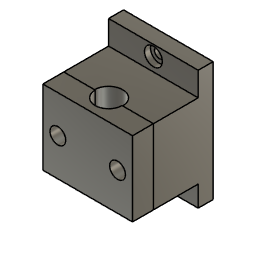
Needle holder v7 (Autodesk Fusion 360 design; units mm, degrees)
Autodesk Fusion 360 part; units mm, degrees
sketch "Sketch1" plane through (0, 0, 0) normal (0, 1, 0) x (1, 0, 0)
  line L0 (0, 0) -> (30, 0)
  line L1 (30, 0) -> (30, -40)
  line L2 (30, -40) -> (0, -40)
  line L3 (0, -40) -> (0, 0)
  circle A0 centre (15, -3.5) radius 1.65
  circle A1 centre (15, -36.5) radius 1.65
  dimension "d1" = 30
  dimension "d2" = 40
  dimension "d3" = 3.3
  dimension "d4" = 3.3
  dimension "d5" = 15
  dimension "d6" = 15
  dimension "d7" = 3.5
  dimension "d8" = 3.5
  constraint horizontal L0
  constraint vertical L1
  constraint horizontal L2
  constraint vertical L3
  constraint coincident L0.start L3.end
  measures "d1" distance of L0.start L0.end
  measures "d2" distance of L0.start L2.end
  measures "d3" diameter of A0
  measures "d4" diameter of A1
  measures "d5" distance of L3 A1.centre
  measures "d6" distance of L3 A0.centre
  measures "d7" distance of L2 A1.centre
  measures "d8" distance of L0 A0.centre
extrude "Extrude1" add sketch "Sketch1" along normal blind 5 makes body 1
sketch "Sketch2" plane through (0, 0, 0) normal (0, -1, 0) x (1, 0, 0)
  circle A0 centre (15, 3.5) radius 1.65
  circle A1 centre (15, 36.5) radius 1.65
  line L0 (30, 40) -> (0, 40)
  line L1 (0, 40) -> (0, 0)
  line L2 (0, 0) -> (30, 0)
  line L3 (30, 0) -> (30, 40)
  line L4 (0, 32) -> (30, 32)
  line L5 (30, 32) -> (30, 7)
  line L6 (30, 7) -> (0, 7)
  line L7 (0, 7) -> (0, 32)
  dimension "d11" = 8
  constraint horizontal L4
  constraint vertical L5
  constraint horizontal L6
  constraint vertical L7
  constraint coincident L3 L5.end
  constraint coincident L1 L4.start
  measures "d11" distance of L0 L4
extrude "Extrude2" add sketch "Sketch2" along normal blind 15 contours L1 L3 L4 L5 L6 L7 bodies 1
sketch "Sketch3" plane through (0, 0, 32) normal (0, 0, 1) x (-1, 0, 0)
  line L0 (-30, 0) -> (0, 0)
  line L1 (0, 0) -> (0, 15)
  line L2 (0, 15) -> (-30, 15)
  line L3 (-30, 15) -> (-30, 0)
  circle A0 centre (-15, 15) radius 4.7245
  dimension "d14" = 9.449
  constraint midpoint L2 A0.centre
  measures "d14" diameter of A0
extrude "Extrude3" cut sketch "Sketch3" against normal blind 25 contours L2 A0 picked at (-16.3012, 14.1129) bodies 1
ref_plane "WorkPlane1" through (15, -7.5, 20.8) normal (0, 0, 1) x (-1, 0, 0)
sketch "Sketch4" plane through (0, 0, 20.8) normal (0, 0, 1) x (1, 0, 0)
  circle A0 centre (15, -15) radius 5.7785
  dimension "d18" = 11.557
  measures "d18" diameter of A0
extrude "Extrude4" cut sketch "Sketch4" against normal blind 11.227 bodies 1
sketch "Sketch5" plane through (0, -15, 0) normal (0, -1, 0) x (1, 0, 0)
  line L0 (19.7245, 20.8) -> (20.7785, 20.8)
  line L1 (20.7785, 20.8) -> (20.7785, 9.573)
  line L2 (20.7785, 9.573) -> (19.7245, 9.573)
  line L3 (19.7245, 9.573) -> (19.7245, 7)
  line L4 (19.7245, 7) -> (30, 7)
  line L5 (30, 7) -> (30, 32)
  line L6 (30, 32) -> (19.7245, 32)
  line L7 (19.7245, 32) -> (19.7245, 20.8)
  circle A0 centre (25, 19.5) radius 2.5
  circle A1 centre (5, 19.5) radius 2.5
  line L8 (10.2755, 32) -> (0, 32)
  line L9 (0, 32) -> (0, 7)
  dimension "d21" = 5
  dimension "d22" = 5
  dimension "d23" = 12.5
  dimension "d24" = 12.5
  dimension "d25" = 5
  dimension "d26" = 5
  measures "d21" diameter of A0
  measures "d22" diameter of A1
  measures "d23" distance of A1.centre L8
  measures "d24" distance of L4 A0.centre
  measures "d25" distance of L5 A0.centre
  measures "d26" distance of A1.centre L9
extrude "Extrude5" cut sketch "Sketch5" against normal blind 5 contours A0 | A1 bodies 1
thread "Thread1" "ISO Metric profile 5.0 M5x0.8 6H" major diameter 5.12 minor diameter 4.234 pitch 0.8 angle 60 modelled right hand crest width 0.2219 on face at (7.4969, -11.6667, 19.3754) crest through (7.117, -14.8, 19.5) on bodies 1
thread "Thread2" "ISO Metric profile 5.0 M5x0.8 6H" major diameter 5.12 minor diameter 4.234 pitch 0.8 angle 60 modelled right hand crest width 0.2219 on face at (27.4969, -11.6667, 19.3754) crest through (27.117, -14.8, 19.5) on bodies 1
box "BoxPrimitive1" add length 25 width 30 height 7 placed x (0, 0, 1) y (-1, 0, 0) z (0, -1, 0) at (30, -15, 12.5) separate body makes body 2
sketch "Sketch9" plane through (0, 0, 37.5) normal (0, 0, 1) x (-1, 0, 0)
  line L0 (-30, 22) -> (-30, 15)
  line L1 (-30, 15) -> (0, 15)
  line L2 (0, 15) -> (0, 22)
  line L3 (0, 22) -> (-30, 22)
  circle A0 centre (-15, 15) radius 4.5
  dimension "d38" = 9
  constraint midpoint L1 A0.centre
  measures "d38" diameter of A0
extrude "Extrude6" cut sketch "Sketch9" against normal blind 25 contours L1 A0 picked at (-16.4501, 15.6657) bodies 2
ref_plane "WorkPlane2" through (15, -18.5, 26.3) normal (0, 0, 1) x (0, 1, 0)
sketch "Sketch10" plane through (0, 0, 26.3) normal (0, 0, 1) x (1, 0, 0)
  circle A0 centre (15, -15) radius 5.7785
  dimension "d42" = 11.557
  measures "d42" diameter of A0
extrude "Extrude7" cut sketch "Sketch10" against normal blind 11.227 bodies 2
sketch "Sketch11" plane through (0, -22, 0) normal (0, -1, 0) x (1, 0, 0)
  line L0 (30, 37.5) -> (0, 37.5)
  line L1 (0, 37.5) -> (0, 12.5)
  line L2 (0, 12.5) -> (30, 12.5)
  line L3 (30, 12.5) -> (30, 37.5)
  circle A0 centre (5, 25) radius 2.65
  circle A1 centre (25, 25) radius 2.65
  dimension "d45" = 5.3
  dimension "d46" = 5.3
  dimension "d47" = 12.5
  dimension "d48" = 12.5
  dimension "d49" = 5
  dimension "d50" = 5
  measures "d45" diameter of A0
  measures "d46" diameter of A1
  measures "d47" distance of L0 A0.centre
  measures "d48" distance of L0 A1.centre
  measures "d49" distance of L1 A0.centre
  measures "d50" distance of L3 A1.centre
extrude "Extrude8" cut sketch "Sketch11" against normal blind 7 contours A0 | A1 bodies 2
sketch "Sketch13" plane through (0, 0, 0) normal (0, -1, 0) x (1, 0, 0)
  line L0 (0, 32) -> (30, 32)
  line L1 (30, 32) -> (30, 40)
  line L2 (30, 40) -> (0, 40)
  line L3 (0, 40) -> (0, 32)
  circle A0 centre (15, 36.5) radius 1.65
  circle A1 centre (15, 36.5) radius 3
  circle A2 centre (15, 3.5) radius 3
  circle A3 centre (15, 3.5) radius 1.65
  constraint concentric A0 A1
  constraint concentric A2 A3
extrude "Extrude10" cut sketch "Sketch13" against normal blind 2 contours A1 | A2 | A3 bodies 1
move_body "Move1" bodies 2 to x (1, 0, 0) y (0, 1, 0) z (0, 0, 1) at (0, 0, -5.5)
named bodies: "base", "cap"
